Autodesk Inventor part; units mm, degrees
(part 2 of 3)
  spline S51 degree 3 poles (0.0984, 19.7366) (0.1649, 19.7419) (0.2979, 19.7525) (0.4939, 19.7932) (0.6876, 19.8429) (0.9422, 19.9224) (1.2539, 20.0412) (1.6171, 20.2089) (1.9698, 20.3977) (2.3118, 20.6053) (2.6441, 20.8281) (2.8566, 20.9892) (2.9629, 21.0697) knots 0 0 0 0 0.062465 0.124964 0.187468 0.249973 0.374966 0.499967 0.624972 0.749981 0.874991 1 1 1 1 construction
  arc A14 (2.9629, 21.0697) -> (2.8257, 22.375) centre (-14, 19.9467) ccw construction
  spline S52 degree 3 poles (2.8257, 22.375) (2.705, 22.4317) (2.4637, 22.545) (2.0923, 22.6939) (1.7146, 22.8258) (1.3304, 22.9372) (0.9402, 23.0257) (0.6106, 23.0771) (0.3451, 23.1019) (0.1453, 23.1102) (-0.055, 23.1093) (-0.1872, 23.092) (-0.2533, 23.0834) knots 0 0 0 0 0.125009 0.250019 0.375028 0.500033 0.625034 0.750027 0.812532 0.875036 0.937535 1 1 1 1 construction
  spline S53 degree 3 poles (-0.2533, 23.0834) (-0.3447, 23.0601) (-0.4818, 23.0252) (-0.668, 22.9946) (-0.8088, 22.9816) (-0.9502, 22.9756) (-1.0916, 22.9828) (-1.2322, 22.9989) (-1.3703, 23.0305) (-1.5044, 23.0763) (-1.6319, 23.1382) (-1.7501, 23.2166) (-1.8562, 23.3108) (-1.9467, 23.42) (-2.0197, 23.5419) (-2.07, 23.6744) (-2.1108, 23.8097) (-2.1574, 23.9432) (-2.1945, 24.08) (-2.2071, 24.2214) (-2.1981, 24.363) (-2.1676, 24.5016) (-2.118, 24.6344) (-2.0513, 24.7595) (-1.9698, 24.8754) (-1.8766, 24.9821) (-1.7723, 25.0778) (-1.6621, 25.1667) (-1.5442, 25.2449) (-1.4226, 25.3172) (-1.254, 25.4019) (-1.1226, 25.4542) (-1.035, 25.4891) knots 0 0 0 0 0.062498 0.093754 0.125008 0.156267 0.187517 0.21877 0.250029 0.281282 0.312529 0.343776 0.37503 0.406277 0.437515 0.468744 0.5 0.531256 0.562485 0.593723 0.62497 0.656224 0.687471 0.718718 0.749971 0.78123 0.812483 0.843733 0.874992 0.906246 0.937502 1 1 1 1 construction
  spline S54 degree 3 poles (-1.035, 25.4891) (-0.9764, 25.521) (-0.8593, 25.5847) (-0.6967, 25.7017) (-0.54, 25.8259) (-0.3398, 26.002) (-0.1033, 26.2373) (0.1603, 26.5383) (0.4057, 26.8542) (0.6337, 27.1829) (0.8467, 27.5217) (0.9753, 27.7552) (1.0396, 27.872) knots 0 0 0 0 0.062465 0.124964 0.187468 0.249973 0.374966 0.499967 0.624972 0.749981 0.874991 1 1 1 1 construction
  arc A15 (1.0396, 27.872) -> (0.3833, 29.0087) centre (-14, 19.9467) ccw construction
  spline S55 degree 3 poles (0.3833, 29.0087) (0.25, 29.0114) (-0.0165, 29.0168) (-0.4164, 29.0017) (-0.815, 28.9686) (-1.2114, 28.9141) (-1.6038, 28.8362) (-1.9258, 28.7491) (-2.1785, 28.6638) (-2.3644, 28.5901) (-2.5469, 28.5079) (-2.6607, 28.4383) (-2.7176, 28.4035) knots 0 0 0 0 0.125009 0.250019 0.375028 0.500033 0.625034 0.750027 0.812532 0.875036 0.937535 1 1 1 1 construction
  spline S56 degree 3 poles (-2.7176, 28.4035) (-2.7916, 28.3451) (-2.9027, 28.2574) (-3.0603, 28.1537) (-3.1837, 28.0846) (-3.3104, 28.0216) (-3.4424, 27.9706) (-3.5775, 27.9282) (-3.7165, 27.9008) (-3.8576, 27.8882) (-3.9993, 27.8929) (-4.1391, 27.9164) (-4.2744, 27.9593) (-4.4015, 28.0223) (-4.5177, 28.1039) (-4.6176, 28.2045) (-4.7099, 28.3115) (-4.8067, 28.4145) (-4.8963, 28.5244) (-4.9653, 28.6485) (-5.0147, 28.7815) (-5.0432, 28.9205) (-5.052, 29.062) (-5.0418, 29.2034) (-5.0145, 29.3424) (-4.9728, 29.4778) (-4.9164, 29.6077) (-4.852, 29.7336) (-4.7761, 29.8531) (-4.6944, 29.9686) (-4.5748, 30.1145) (-4.476, 30.2158) (-4.4102, 30.2833) knots 0 0 0 0 0.062498 0.093754 0.125008 0.156267 0.187517 0.21877 0.250029 0.281282 0.312529 0.343776 0.37503 0.406277 0.437515 0.468744 0.5 0.531256 0.562485 0.593723 0.62497 0.656224 0.687471 0.718718 0.749971 0.78123 0.812483 0.843733 0.874992 0.906246 0.937502 1 1 1 1 construction
  spline S57 degree 3 poles (-4.4102, 30.2833) (-4.3696, 30.3362) (-4.2885, 30.4421) (-4.1876, 30.6151) (-4.095, 30.7923) (-3.9837, 31.0346) (-3.8634, 31.3457) (-3.745, 31.7279) (-3.6493, 32.1164) (-3.5747, 32.5094) (-3.5179, 32.9054) (-3.4954, 33.1711) (-3.4842, 33.304) knots 0 0 0 0 0.062465 0.124964 0.187468 0.249973 0.374966 0.499967 0.624972 0.749981 0.874991 1 1 1 1 construction
  arc A16 (-3.4842, 33.304) -> (-4.546, 34.0754) centre (-14, 19.9467) ccw construction
  spline S58 degree 3 poles (-4.546, 34.0754) (-4.6689, 34.0237) (-4.9146, 33.9202) (-5.2737, 33.7438) (-5.6245, 33.5514) (-5.9644, 33.3404) (-6.2912, 33.1097) (-6.55, 32.8991) (-6.7461, 32.7184) (-6.8859, 32.5755) (-7.0193, 32.4261) (-7.0949, 32.3162) (-7.1327, 32.2613) knots 0 0 0 0 0.125009 0.250019 0.375028 0.500033 0.625034 0.750027 0.812532 0.875036 0.937535 1 1 1 1 construction
  spline S59 degree 3 poles (-7.1327, 32.2613) (-7.1766, 32.1779) (-7.2424, 32.0526) (-7.3442, 31.8938) (-7.4288, 31.7804) (-7.5189, 31.6713) (-7.6188, 31.5711) (-7.7249, 31.4773) (-7.8408, 31.3958) (-7.9646, 31.3269) (-8.0959, 31.2736) (-8.2332, 31.2381) (-8.3742, 31.2223) (-8.516, 31.2282) (-8.6553, 31.2555) (-8.7875, 31.3067) (-8.9154, 31.3669) (-9.0457, 31.4216) (-9.1722, 31.4856) (-9.2858, 31.5709) (-9.3849, 31.6723) (-9.4676, 31.7877) (-9.5331, 31.9134) (-9.5814, 32.0467) (-9.6129, 32.1848) (-9.6299, 32.3255) (-9.6312, 32.467) (-9.6236, 32.6084) (-9.6028, 32.7484) (-9.5752, 32.8871) (-9.5253, 33.069) (-9.4762, 33.2017) (-9.4436, 33.2902) knots 0 0 0 0 0.062498 0.093754 0.125008 0.156267 0.187517 0.21877 0.250029 0.281282 0.312529 0.343776 0.37503 0.406277 0.437515 0.468744 0.5 0.531256 0.562485 0.593723 0.62497 0.656224 0.687471 0.718718 0.749971 0.78123 0.812483 0.843733 0.874992 0.906246 0.937502 1 1 1 1 construction
  spline S60 degree 3 poles (-9.4436, 33.2902) (-9.428, 33.355) (-9.397, 33.4847) (-9.3752, 33.6838) (-9.3626, 33.8833) (-9.3595, 34.15) (-9.3762, 34.4832) (-9.4234, 34.8805) (-9.494, 35.2743) (-9.5857, 35.6636) (-9.695, 36.0485) (-9.7825, 36.3004) (-9.8262, 36.4263) knots 0 0 0 0 0.062465 0.124964 0.187468 0.249973 0.374966 0.499967 0.624972 0.749981 0.874991 1 1 1 1 construction
  arc A17 (-9.8262, 36.4263) -> (-11.11, 36.6992) centre (-14, 19.9467) ccw construction
  spline S61 degree 3 poles (-11.11, 36.6992) (-11.2012, 36.602) (-11.3836, 36.4075) (-11.64, 36.1003) (-11.8821, 35.7819) (-12.1068, 35.4508) (-12.3116, 35.1071) (-12.4623, 34.8095) (-12.5679, 34.5647) (-12.6376, 34.3772) (-12.6986, 34.1865) (-12.723, 34.0554) (-12.7352, 33.9898) knots 0 0 0 0 0.125009 0.250019 0.375028 0.500033 0.625034 0.750027 0.812532 0.875036 0.937535 1 1 1 1 construction
  spline S62 degree 3 poles (-12.7352, 33.9898) (-12.7413, 33.8958) (-12.7505, 33.7546) (-12.7789, 33.5681) (-12.8101, 33.4301) (-12.8481, 33.2938) (-12.8986, 33.1615) (-12.9574, 33.0328) (-13.0301, 32.9112) (-13.1151, 32.7978) (-13.2134, 32.6957) (-13.3244, 32.6075) (-13.4468, 32.5357) (-13.5787, 32.4834) (-13.7171, 32.4516) (-13.8587, 32.4447) (-14, 32.4477) (-14.1413, 32.4447) (-14.2829, 32.4516) (-14.4213, 32.4834) (-14.5532, 32.5357) (-14.6756, 32.6075) (-14.7866, 32.6957) (-14.8849, 32.7978) (-14.9699, 32.9112) (-15.0426, 33.0328) (-15.1014, 33.1615) (-15.1519, 33.2938) (-15.1899, 33.4301) (-15.2211, 33.5681) (-15.2495, 33.7546) (-15.2587, 33.8958) (-15.2648, 33.9898) knots 0 0 0 0 0.062498 0.093754 0.125008 0.156267 0.187517 0.21877 0.250029 0.281282 0.312529 0.343776 0.37503 0.406277 0.437515 0.468744 0.5 0.531256 0.562485 0.593723 0.62497 0.656224 0.687471 0.718718 0.749971 0.78123 0.812483 0.843733 0.874992 0.906246 0.937502 1 1 1 1 construction
  spline S63 degree 3 poles (-15.2648, 33.9898) (-15.277, 34.0554) (-15.3014, 34.1865) (-15.3624, 34.3772) (-15.4321, 34.5647) (-15.5377, 34.8095) (-15.6884, 35.1071) (-15.8932, 35.4508) (-16.1179, 35.7819) (-16.36, 36.1003) (-16.6164, 36.4075) (-16.7988, 36.602) (-16.89, 36.6992) knots 0 0 0 0 0.062465 0.124964 0.187468 0.249973 0.374966 0.499967 0.624972 0.749981 0.874991 1 1 1 1 construction
  arc A18 (-16.89, 36.6992) -> (-18.1738, 36.4263) centre (-14, 19.9467) ccw construction
  circle A19 centre (-14, 19.9467) radius 1.1 construction
  spline S64 degree 3 poles (-41.4547, 4.7129) (-41.4384, 4.8452) (-41.4058, 5.1098) (-41.3799, 5.5091) (-41.3721, 5.9091) (-41.3859, 6.3089) (-41.4232, 6.7073) (-41.477, 7.0365) (-41.5361, 7.2965) (-41.5904, 7.489) (-41.6536, 7.679) (-41.7112, 7.7993) (-41.74, 7.8594) knots 0 0 0 0 0.125009 0.250019 0.375028 0.500033 0.625034 0.750027 0.812532 0.875036 0.937535 1 1 1 1 construction
  spline S65 degree 3 poles (-41.74, 7.8594) (-41.7905, 7.939) (-41.8663, 8.0584) (-41.9534, 8.2258) (-42.0096, 8.3556) (-42.0593, 8.4881) (-42.0965, 8.6247) (-42.125, 8.7634) (-42.1379, 8.9044) (-42.1361, 9.0461) (-42.117, 9.1866) (-42.0793, 9.3233) (-42.0228, 9.4534) (-41.9472, 9.5734) (-41.8541, 9.6807) (-41.7438, 9.7698) (-41.6279, 9.8507) (-41.5156, 9.9365) (-41.3972, 10.0144) (-41.2666, 10.0704) (-41.1293, 10.1059) (-40.9881, 10.1201) (-40.8464, 10.1143) (-40.7068, 10.0898) (-40.5713, 10.0484) (-40.4409, 9.9931) (-40.3175, 9.9238) (-40.1987, 9.8467) (-40.0876, 9.759) (-39.9811, 9.666) (-39.8482, 9.5321) (-39.7575, 9.4235) (-39.6971, 9.3511) knots 0 0 0 0 0.062498 0.093754 0.125008 0.156267 0.187517 0.21877 0.250029 0.281282 0.312529 0.343776 0.37503 0.406277 0.437515 0.468744 0.5 0.531256 0.562485 0.593723 0.62497 0.656224 0.687471 0.718718 0.749971 0.78123 0.812483 0.843733 0.874992 0.906246 0.937502 1 1 1 1 construction
  spline S66 degree 3 poles (-39.6971, 9.3511) (-39.6486, 9.3054) (-39.5515, 9.2139) (-39.3897, 9.0958) (-39.223, 8.9856) (-38.9932, 8.8501) (-38.6961, 8.6987) (-38.328, 8.5418) (-37.9513, 8.4069) (-37.568, 8.2926) (-37.1798, 8.1957) (-36.9178, 8.1462) (-36.7868, 8.1214) knots 0 0 0 0 0.062465 0.124964 0.187468 0.249973 0.374966 0.499967 0.624972 0.749981 0.874991 1 1 1 1 construction
  arc A20 (-36.7868, 8.1214) -> (-35.9109, 9.0989) centre (-49, 19.9467) ccw construction
  spline S67 degree 3 poles (-35.9109, 9.0989) (-35.9498, 9.2264) (-36.0277, 9.4814) (-36.1664, 9.8567) (-36.322, 10.2252) (-36.4972, 10.5849) (-36.6933, 10.9336) (-36.8763, 11.2125) (-37.0361, 11.426) (-37.1639, 11.5798) (-37.299, 11.7277) (-37.4005, 11.8141) (-37.4513, 11.8573) knots 0 0 0 0 0.125009 0.250019 0.375028 0.500033 0.625034 0.750027 0.812532 0.875036 0.937535 1 1 1 1 construction
  spline S68 degree 3 poles (-37.4513, 11.8573) (-37.5298, 11.9095) (-37.6477, 11.9877) (-37.7953, 12.1053) (-37.8994, 12.201) (-37.9987, 12.3018) (-38.0883, 12.4114) (-38.1707, 12.5265) (-38.2399, 12.6501) (-38.2959, 12.7803) (-38.3355, 12.9164) (-38.3567, 13.0566) (-38.358, 13.1985) (-38.3377, 13.3389) (-38.2963, 13.4748) (-38.2319, 13.601) (-38.1589, 13.7221) (-38.0912, 13.8461) (-38.0146, 13.9654) (-37.9182, 14.0697) (-37.8071, 14.158) (-37.6839, 14.2284) (-37.5522, 14.2807) (-37.4146, 14.3151) (-37.274, 14.3324) (-37.1324, 14.3349) (-36.9914, 14.3218) (-36.8516, 14.2997) (-36.7145, 14.2648) (-36.5793, 14.2231) (-36.4034, 14.1549) (-36.2764, 14.0925) (-36.1918, 14.051) knots 0 0 0 0 0.062498 0.093754 0.125008 0.156267 0.187517 0.21877 0.250029 0.281282 0.312529 0.343776 0.37503 0.406277 0.437515 0.468744 0.5 0.531256 0.562485 0.593723 0.62497 0.656224 0.687471 0.718718 0.749971 0.78123 0.812483 0.843733 0.874992 0.906246 0.937502 1 1 1 1 construction
  spline S69 degree 3 poles (-36.1918, 14.051) (-36.1288, 14.0289) (-36.003, 13.9848) (-35.8072, 13.9428) (-35.61, 13.9099) (-35.345, 13.8796) (-35.0119, 13.8621) (-34.6118, 13.8685) (-34.2129, 13.8985) (-33.8162, 13.95) (-33.4221, 14.0193) (-33.1626, 14.0806) (-33.0329, 14.1113) knots 0 0 0 0 0.062465 0.124964 0.187468 0.249973 0.374966 0.499967 0.624972 0.749981 0.874991 1 1 1 1 construction
  arc A21 (-33.0329, 14.1113) -> (-32.6303, 15.3605) centre (-49, 19.9467) ccw construction
  spline S70 degree 3 poles (-32.6303, 15.3605) (-32.7177, 15.4612) (-32.8926, 15.6625) (-33.172, 15.9489) (-33.464, 16.2223) (-33.7703, 16.4796) (-34.0914, 16.7184) (-34.372, 16.8987) (-34.6048, 17.0288) (-34.7841, 17.1173) (-34.9676, 17.1975) (-35.0955, 17.2352) (-35.1595, 17.254) knots 0 0 0 0 0.125009 0.250019 0.375028 0.500033 0.625034 0.750027 0.812532 0.875036 0.937535 1 1 1 1 construction
  spline S71 degree 3 poles (-35.1595, 17.254) (-35.2525, 17.2697) (-35.3919, 17.2932) (-35.5746, 17.3405) (-35.7087, 17.3857) (-35.8404, 17.4374) (-35.9668, 17.5011) (-36.0889, 17.5727) (-36.2024, 17.6575) (-36.3065, 17.7536) (-36.398, 17.8619) (-36.4744, 17.9813) (-36.5333, 18.1104) (-36.5719, 18.2469) (-36.5893, 18.3879) (-36.5818, 18.5294) (-36.5644, 18.6697) (-36.553, 18.8105) (-36.5316, 18.9507) (-36.4858, 19.0851) (-36.4203, 19.211) (-36.3364, 19.3254) (-36.2373, 19.4268) (-36.1257, 19.5142) (-36.0043, 19.5872) (-35.8759, 19.6471) (-35.7418, 19.6924) (-35.6051, 19.7291) (-35.4656, 19.753) (-35.3251, 19.7699) (-35.1367, 19.7791) (-34.9953, 19.7738) (-34.9011, 19.7703) knots 0 0 0 0 0.062498 0.093754 0.125008 0.156267 0.187517 0.21877 0.250029 0.281282 0.312529 0.343776 0.37503 0.406277 0.437515 0.468744 0.5 0.531256 0.562485 0.593723 0.62497 0.656224 0.687471 0.718718 0.749971 0.78123 0.812483 0.843733 0.874992 0.906246 0.937502 1 1 1 1 construction
  spline S72 degree 3 poles (-34.9011, 19.7703) (-34.8347, 19.7757) (-34.7017, 19.7866) (-34.5057, 19.8279) (-34.3122, 19.878) (-34.0578, 19.9581) (-33.7464, 20.0776) (-33.3836, 20.2462) (-33.0313, 20.4359) (-32.6898, 20.6442) (-32.358, 20.8679) (-32.1459, 21.0294) (-32.0399, 21.1102) knots 0 0 0 0 0.062465 0.124964 0.187468 0.249973 0.374966 0.499967 0.624972 0.749981 0.874991 1 1 1 1 construction
  arc A22 (-32.0399, 21.1102) -> (-32.1802, 22.4152) centre (-49, 19.9467) ccw construction
  spline S73 degree 3 poles (-32.1802, 22.4152) (-32.301, 22.4716) (-32.5426, 22.5844) (-32.9143, 22.7323) (-33.2923, 22.8633) (-33.6768, 22.9738) (-34.0672, 23.0614) (-34.3969, 23.112) (-34.6625, 23.1362) (-34.8623, 23.144) (-35.0626, 23.1426) (-35.1948, 23.125) (-35.2609, 23.1162) knots 0 0 0 0 0.125009 0.250019 0.375028 0.500033 0.625034 0.750027 0.812532 0.875036 0.937535 1 1 1 1 construction
  spline S74 degree 3 poles (-35.2609, 23.1162) (-35.3522, 23.0927) (-35.4892, 23.0575) (-35.6753, 23.0265) (-35.8161, 23.0131) (-35.9575, 23.0068) (-36.0989, 23.0136) (-36.2395, 23.0294) (-36.3777, 23.0606) (-36.5119, 23.1062) (-36.6395, 23.1678) (-36.7579, 23.2458) (-36.8643, 23.3398) (-36.955, 23.4488) (-37.0283, 23.5705) (-37.079, 23.7029) (-37.1201, 23.8381) (-37.167, 23.9714) (-37.2044, 24.1082) (-37.2173, 24.2496) (-37.2087, 24.3912) (-37.1785, 24.5299) (-37.1293, 24.6628) (-37.0628, 24.788) (-36.9816, 24.9041) (-36.8886, 25.0111) (-36.7846, 25.107) (-36.6746, 25.1961) (-36.5569, 25.2747) (-36.4355, 25.3473) (-36.2671, 25.4323) (-36.1358, 25.485) (-36.0483, 25.5201) knots 0 0 0 0 0.062498 0.093754 0.125008 0.156267 0.187517 0.21877 0.250029 0.281282 0.312529 0.343776 0.37503 0.406277 0.437515 0.468744 0.5 0.531256 0.562485 0.593723 0.62497 0.656224 0.687471 0.718718 0.749971 0.78123 0.812483 0.843733 0.874992 0.906246 0.937502 1 1 1 1 construction
  spline S75 degree 3 poles (-36.0483, 25.5201) (-35.9898, 25.5521) (-35.8728, 25.6161) (-35.7105, 25.7335) (-35.5541, 25.858) (-35.3543, 26.0346) (-35.1184, 26.2705) (-34.8555, 26.5721) (-34.6108, 26.8886) (-34.3836, 27.2179) (-34.1715, 27.5571) (-34.0434, 27.791) (-33.9794, 27.9079) knots 0 0 0 0 0.062465 0.124964 0.187468 0.249973 0.374966 0.499967 0.624972 0.749981 0.874991 1 1 1 1 construction
  arc A23 (-33.9794, 27.9079) -> (-34.6384, 29.043) centre (-49, 19.9467) ccw construction
  spline S76 degree 3 poles (-34.6384, 29.043) (-34.7717, 29.0454) (-35.0383, 29.0501) (-35.438, 29.0341) (-35.8366, 29.0001) (-36.2328, 28.9446) (-36.6251, 28.8658) (-36.9469, 28.7779) (-37.1993, 28.692) (-37.385, 28.6179) (-37.5674, 28.5352) (-37.681, 28.4653) (-37.7378, 28.4304) knots 0 0 0 0 0.125009 0.250019 0.375028 0.500033 0.625034 0.750027 0.812532 0.875036 0.937535 1 1 1 1 construction
  spline S77 degree 3 poles (-37.7378, 28.4304) (-37.8117, 28.3718) (-37.9225, 28.2839) (-38.0799, 28.1798) (-38.2032, 28.1104) (-38.3297, 28.0471) (-38.4616, 27.9958) (-38.5966, 27.953) (-38.7355, 27.9254) (-38.8766, 27.9124) (-39.0183, 27.9168) (-39.1582, 27.9399) (-39.2935, 27.9825) (-39.4208, 28.0452) (-39.5372, 28.1265) (-39.6374, 28.2268) (-39.73, 28.3337) (-39.827, 28.4364) (-39.9168, 28.5461) (-39.9861, 28.67) (-40.0358, 28.8029) (-40.0647, 28.9418) (-40.0738, 29.0833) (-40.064, 29.2248) (-40.037, 29.3638) (-39.9956, 29.4993) (-39.9396, 29.6293) (-39.8754, 29.7555) (-39.7998, 29.8751) (-39.7184, 29.9908) (-39.5991, 30.137) (-39.5006, 30.2385) (-39.4349, 30.3062) knots 0 0 0 0 0.062498 0.093754 0.125008 0.156267 0.187517 0.21877 0.250029 0.281282 0.312529 0.343776 0.37503 0.406277 0.437515 0.468744 0.5 0.531256 0.562485 0.593723 0.62497 0.656224 0.687471 0.718718 0.749971 0.78123 0.812483 0.843733 0.874992 0.906246 0.937502 1 1 1 1 construction
  spline S78 degree 3 poles (-39.4349, 30.3062) (-39.3945, 30.3592) (-39.3136, 30.4653) (-39.2132, 30.6385) (-39.1209, 30.8159) (-39.0102, 31.0585) (-38.8907, 31.3699) (-38.7731, 31.7524) (-38.6784, 32.1411) (-38.6048, 32.5343) (-38.5489, 32.9305) (-38.5271, 33.1962) (-38.5161, 33.3291) knots 0 0 0 0 0.062465 0.124964 0.187468 0.249973 0.374966 0.499967 0.624972 0.749981 0.874991 1 1 1 1 construction
  arc A24 (-38.5161, 33.3291) -> (-39.5798, 34.098) centre (-49, 19.9467) ccw construction
  spline S79 degree 3 poles (-39.5798, 34.098) (-39.7025, 34.046) (-39.948, 33.9419) (-40.3067, 33.7646) (-40.657, 33.5714) (-40.9964, 33.3595) (-41.3227, 33.128) (-41.5809, 32.9169) (-41.7766, 32.7357) (-41.9161, 32.5925) (-42.0491, 32.4427) (-42.1245, 32.3327) (-42.1621, 32.2777) knots 0 0 0 0 0.125009 0.250019 0.375028 0.500033 0.625034 0.750027 0.812532 0.875036 0.937535 1 1 1 1 construction
  spline S80 degree 3 poles (-42.1621, 32.2777) (-42.2058, 32.1941) (-42.2713, 32.0687) (-42.3727, 31.9096) (-42.4571, 31.7961) (-42.547, 31.6868) (-42.6466, 31.5863) (-42.7525, 31.4923) (-42.8682, 31.4105) (-42.9918, 31.3413) (-43.123, 31.2876) (-43.2602, 31.2519) (-43.4012, 31.2357) (-43.5429, 31.2412) (-43.6824, 31.2682) (-43.8147, 31.3191) (-43.9427, 31.379) (-44.0731, 31.4334) (-44.1998, 31.4971) (-44.3135, 31.5821) (-44.413, 31.6833) (-44.4959, 31.7985) (-44.5617, 31.9241) (-44.6103, 32.0572) (-44.6422, 32.1953) (-44.6595, 32.3359) (-44.6612, 32.4774) (-44.6538, 32.6188) (-44.6334, 32.7588) (-44.6061, 32.8976) (-44.5566, 33.0797) (-44.5079, 33.2125) (-44.4754, 33.301) knots 0 0 0 0 0.062498 0.093754 0.125008 0.156267 0.187517 0.21877 0.250029 0.281282 0.312529 0.343776 0.37503 0.406277 0.437515 0.468744 0.5 0.531256 0.562485 0.593723 0.62497 0.656224 0.687471 0.718718 0.749971 0.78123 0.812483 0.843733 0.874992 0.906246 0.937502 1 1 1 1 construction
  spline S81 degree 3 poles (-44.4754, 33.301) (-44.4601, 33.3659) (-44.4294, 33.4957) (-44.408, 33.6948) (-44.3959, 33.8944) (-44.3935, 34.1611) (-44.4109, 34.4942) (-44.4591, 34.8913) (-44.5306, 35.285) (-44.6233, 35.6741) (-44.7334, 36.0588) (-44.8216, 36.3104) (-44.8656, 36.4363) knots 0 0 0 0 0.062465 0.124964 0.187468 0.249973 0.374966 0.499967 0.624972 0.749981 0.874991 1 1 1 1 construction
  arc A25 (-44.8656, 36.4363) -> (-46.1501, 36.7061) centre (-49, 19.9467) ccw construction
  spline S82 degree 3 poles (-46.1501, 36.7061) (-46.241, 36.6086) (-46.423, 36.4137) (-46.6786, 36.1059) (-46.92, 35.7869) (-47.1438, 35.4553) (-47.3478, 35.1111) (-47.4978, 34.8132) (-47.6028, 34.568) (-47.6721, 34.3805) (-47.7326, 34.1896) (-47.7567, 34.0584) (-47.7688, 33.9928) knots 0 0 0 0 0.125009 0.250019 0.375028 0.500033 0.625034 0.750027 0.812532 0.875036 0.937535 1 1 1 1 construction
  spline S83 degree 3 poles (-47.7688, 33.9928) (-47.7747, 33.8987) (-47.7835, 33.7575) (-47.8115, 33.5709) (-47.8423, 33.4329) (-47.88, 33.2965) (-47.9301, 33.1641) (-47.9886, 33.0352) (-48.0611, 32.9134) (-48.1458, 32.7999) (-48.2439, 32.6975) (-48.3547, 32.6091) (-48.4769, 32.537) (-48.6086, 32.4844) (-48.747, 32.4523) (-48.8886, 32.445) (-49.0299, 32.4476) (-49.1712, 32.4443) (-49.3128, 32.4509) (-49.4513, 32.4823) (-49.5833, 32.5343) (-49.7058, 32.6058) (-49.8171, 32.6938) (-49.9156, 32.7957) (-50.0009, 32.9088) (-50.0739, 33.0302) (-50.133, 33.1589) (-50.1838, 33.291) (-50.2221, 33.4272) (-50.2536, 33.5651) (-50.2825, 33.7516) (-50.292, 33.8927) (-50.2983, 33.9868) knots 0 0 0 0 0.062498 0.093754 0.125008 0.156267 0.187517 0.21877 0.250029 0.281282 0.312529 0.343776 0.37503 0.406277 0.437515 0.468744 0.5 0.531256 0.562485 0.593723 0.62497 0.656224 0.687471 0.718718 0.749971 0.78123 0.812483 0.843733 0.874992 0.906246 0.937502 1 1 1 1 construction
  spline S84 degree 3 poles (-50.2983, 33.9868) (-50.3107, 34.0523) (-50.3354, 34.1834) (-50.3969, 34.3739) (-50.467, 34.5612) (-50.5732, 34.8058) (-50.7246, 35.103) (-50.9302, 35.4463) (-51.1557, 35.7768) (-51.3986, 36.0946) (-51.6557, 36.4012) (-51.8385, 36.5952) (-51.93, 36.6923) knots 0 0 0 0 0.062465 0.124964 0.187468 0.249973 0.374966 0.499967 0.624972 0.749981 0.874991 1 1 1 1 construction
  arc A26 (-51.93, 36.6923) -> (-53.2131, 36.4163) centre (-49, 19.9467) ccw construction
  spline S85 degree 3 poles (-53.2131, 36.4163) (-53.2566, 36.2903) (-53.3435, 36.0382) (-53.4518, 35.653) (-53.5426, 35.2635) (-53.6122, 34.8695) (-53.6586, 34.4721) (-53.6744, 34.1389) (-53.6707, 33.8722) (-53.6576, 33.6727) (-53.6353, 33.4737) (-53.604, 33.3441) (-53.5883, 33.2793) knots 0 0 0 0 0.125009 0.250019 0.375028 0.500033 0.625034 0.750027 0.812532 0.875036 0.937535 1 1 1 1 construction
  spline S86 degree 3 poles (-53.5883, 33.2793) (-53.5554, 33.1909) (-53.5061, 33.0583) (-53.4557, 32.8765) (-53.4278, 32.7378) (-53.4067, 32.5979) (-53.3987, 32.4566) (-53.3997, 32.315) (-53.4163, 32.1743) (-53.4475, 32.0361) (-53.4955, 31.9027) (-53.5607, 31.7768) (-53.6431, 31.6613) (-53.742, 31.5596) (-53.8554, 31.474) (-53.9817, 31.4098) (-54.1119, 31.3547) (-54.2396, 31.2942) (-54.3717, 31.2427) (-54.511, 31.215) (-54.6527, 31.2089) (-54.7937, 31.2243) (-54.9311, 31.2594) (-55.0626, 31.3124) (-55.1865, 31.3811) (-55.3026, 31.4623) (-55.4089, 31.5558) (-55.5091, 31.6558) (-55.5995, 31.7647) (-55.6843, 31.8778) (-55.7865, 32.0365) (-55.8526, 32.1615) (-55.8967, 32.2449) knots 0 0 0 0 0.062498 0.093754 0.125008 0.156267 0.187517 0.21877 0.250029 0.281282 0.312529 0.343776 0.37503 0.406277 0.437515 0.468744 0.5 0.531256 0.562485 0.593723 0.62497 0.656224 0.687471 0.718718 0.749971 0.78123 0.812483 0.843733 0.874992 0.906246 0.937502 1 1 1 1 construction
  spline S87 degree 3 poles (-55.8967, 32.2449) (-55.9346, 32.2997) (-56.0105, 32.4094) (-56.1442, 32.5585) (-56.2844, 32.701) (-56.481, 32.8813) (-56.7402, 33.0912) (-57.0676, 33.3212) (-57.408, 33.5314) (-57.7592, 33.7229) (-58.1187, 33.8985) (-58.3647, 34.0014) (-58.4877, 34.0528) knots 0 0 0 0 0.062465 0.124964 0.187468 0.249973 0.374966 0.499967 0.624972 0.749981 0.874991 1 1 1 1 construction
  arc A27 (-58.4877, 34.0528) -> (-59.5477, 33.2788) centre (-49, 19.9467) ccw construction
  spline S88 degree 3 poles (-59.5477, 33.2788) (-59.5361, 33.146) (-59.513, 32.8804) (-59.4553, 32.4845) (-59.3798, 32.0916) (-59.2831, 31.7034) (-59.1638, 31.3215) (-59.0428, 31.0107) (-58.9309, 30.7686) (-58.8378, 30.5916) (-58.7365, 30.4189) (-58.6551, 30.3132) (-58.6145, 30.2604) knots 0 0 0 0 0.125009 0.250019 0.375028 0.500033 0.625034 0.750027 0.812532 0.875036 0.937535 1 1 1 1 construction
  spline S89 degree 3 poles (-58.6145, 30.2604) (-58.5485, 30.193) (-58.4495, 30.092) (-58.3295, 29.9463) (-58.2476, 29.831) (-58.1714, 29.7118) (-58.1066, 29.5859) (-58.0499, 29.4562) (-58.0079, 29.3209) (-57.9803, 29.182) (-57.9698, 29.0406) (-57.9782, 28.899) (-58.0064, 28.76) (-58.0554, 28.6269) (-58.1242, 28.5026) (-58.2135, 28.3925) (-58.31, 28.2893) (-58.4021, 28.182) (-58.5018, 28.0812) (-58.6178, 27.9993) (-58.7447, 27.936) (-58.8799, 27.8928) (-59.0197, 27.869) (-59.1613, 27.8639) (-59.3025, 27.8762) (-59.4416, 27.9032) (-59.5767, 27.9454) (-59.7088, 27.996) (-59.8357, 28.0587) (-59.9593, 28.1276) (-60.1172, 28.2309) (-60.2284, 28.3183) (-60.3026, 28.3765) knots 0 0 0 0 0.062498 0.093754 0.125008 0.156267 0.187517 0.21877 0.250029 0.281282 0.312529 0.343776 0.37503 0.406277 0.437515 0.468744 0.5 0.531256 0.562485 0.593723 0.62497 0.656224 0.687471 0.718718 0.749971 0.78123 0.812483 0.843733 0.874992 0.906246 0.937502 1 1 1 1 construction
  spline S90 degree 3 poles (-60.3026, 28.3765) (-60.3595, 28.4112) (-60.4735, 28.4805) (-60.6563, 28.5623) (-60.8423, 28.6355) (-61.0952, 28.7203) (-61.4174, 28.8066) (-61.81, 28.8835) (-62.2065, 28.9371) (-62.6052, 28.9692) (-63.0051, 28.9833) (-63.2717, 28.9773) (-63.4049, 28.9743) knots 0 0 0 0 0.062465 0.124964 0.187468 0.249973 0.374966 0.499967 0.624972 0.749981 0.874991 1 1 1 1 construction
  arc A28 (-63.4049, 28.9743) -> (-64.0585, 27.8361) centre (-49, 19.9467) ccw construction
  spline S91 degree 3 poles (-64.0585, 27.8361) (-63.9939, 27.7194) (-63.8647, 27.4862) (-63.6509, 27.148) (-63.4222, 26.8198) (-63.176, 26.5044) (-62.9117, 26.2041) (-62.6747, 25.9694) (-62.474, 25.7937) (-62.317, 25.6699) (-62.1542, 25.5533) (-62.0369, 25.4898) (-61.9782, 25.4581) knots 0 0 0 0 0.125009 0.250019 0.375028 0.500033 0.625034 0.750027 0.812532 0.875036 0.937535 1 1 1 1 construction
  spline S92 degree 3 poles (-61.9782, 25.4581) (-61.8905, 25.4234) (-61.759, 25.3714) (-61.5902, 25.2872) (-61.4684, 25.2152) (-61.3503, 25.1372) (-61.2399, 25.0486) (-61.1354, 24.9531) (-61.042, 24.8466) (-60.9602, 24.7309) (-60.8931, 24.606) (-60.8432, 24.4733) (-60.8125, 24.3348) (-60.8031, 24.1932) (-60.8154, 24.0517) (-60.8521, 23.9148) (-60.8984, 23.7813) (-60.9388, 23.6459) (-60.9889, 23.5133) (-61.0616, 23.3912) (-61.1518, 23.2818) (-61.2577, 23.1873) (-61.3757, 23.1087) (-61.5031, 23.0465) (-61.637, 23.0003) (-61.7751, 22.9684) (-61.9157, 22.9519) (-62.057, 22.9444) (-62.1984, 22.9501) (-62.3393, 22.9627) (-62.5255, 22.9929) (-62.6627, 23.0275) (-62.7541, 23.0505) knots 0 0 0 0 0.062498 0.093754 0.125008 0.156267 0.187517 0.21877 0.250029 0.281282 0.312529 0.343776 0.37503 0.406277 0.437515 0.468744 0.5 0.531256 0.562485 0.593723 0.62497 0.656224 0.687471 0.718718 0.749971 0.78123 0.812483 0.843733 0.874992 0.906246 0.937502 1 1 1 1 construction
  spline S93 degree 3 poles (-62.7541, 23.0505) (-62.8203, 23.059) (-62.9525, 23.076) (-63.1528, 23.0764) (-63.3526, 23.0676) (-63.618, 23.0422) (-63.9475, 22.99) (-64.3375, 22.9005) (-64.7215, 22.7883) (-65.0988, 22.6554) (-65.4698, 22.5057) (-65.7109, 22.3918) (-65.8314, 22.3348) knots 0 0 0 0 0.062465 0.124964 0.187468 0.249973 0.374966 0.499967 0.624972 0.749981 0.874991 1 1 1 1 construction
  arc A29 (-65.8314, 22.3348) -> (-65.9655, 21.0292) centre (-49, 19.9467) ccw construction
  spline S94 degree 3 poles (-65.9655, 21.0292) (-65.8591, 20.9489) (-65.6462, 20.7883) (-65.3133, 20.5663) (-64.9709, 20.3596) (-64.6177, 20.1716) (-64.254, 20.0047) (-63.9421, 19.8867) (-63.6873, 19.8078) (-63.4935, 19.7586) (-63.2973, 19.7183) (-63.1644, 19.708) (-63.0979, 19.7029) knots 0 0 0 0 0.125009 0.250019 0.375028 0.500033 0.625034 0.750027 0.812532 0.875036 0.937535 1 1 1 1 construction
  spline S95 degree 3 poles (-63.0979, 19.7029) (-63.0037, 19.7069) (-62.8624, 19.7129) (-62.6739, 19.7046) (-62.5333, 19.6883) (-62.3937, 19.6651) (-62.2569, 19.6291) (-62.1226, 19.5844) (-61.9939, 19.5251) (-61.8721, 19.4527) (-61.7601, 19.3658) (-61.6605, 19.2649) (-61.576, 19.1509) (-61.5099, 19.0254) (-61.4635, 18.8911) (-61.4415, 18.7511) (-61.4294, 18.6103) (-61.4113, 18.4701) (-61.4031, 18.3286) (-61.4198, 18.1875) (-61.4577, 18.0508) (-61.516, 17.9215) (-61.5919, 17.8017) (-61.6829, 17.693) (-61.7865, 17.5964) (-61.8996, 17.5111) (-62.0214, 17.4388) (-62.1475, 17.3745) (-62.2789, 17.3222) (-62.4128, 17.2764) (-62.5952, 17.2282) (-62.7346, 17.204) (-62.8275, 17.1879) knots 0 0 0 0 0.062498 0.093754 0.125008 0.156267 0.187517 0.21877 0.250029 0.281282 0.312529 0.343776 0.37503 0.406277 0.437515 0.468744 0.5 0.531256 0.562485 0.593723 0.62497 0.656224 0.687471 0.718718 0.749971 0.78123 0.812483 0.843733 0.874992 0.906246 0.937502 1 1 1 1 construction
  spline S96 degree 3 poles (-62.8275, 17.1879) (-62.8913, 17.1687) (-63.0191, 17.1304) (-63.2022, 17.0494) (-63.3811, 16.9601) (-63.6133, 16.8289) (-63.893, 16.6472) (-64.2129, 16.4069) (-64.5181, 16.1481) (-64.8087, 15.8733) (-65.0868, 15.5856) (-65.2607, 15.3834) (-65.3476, 15.2824) knots 0 0 0 0 0.062465 0.124964 0.187468 0.249973 0.374966 0.499967 0.624972 0.749981 0.874991 1 1 1 1 construction
  arc A30 (-65.3476, 15.2824) -> (-64.939, 14.0351) centre (-49, 19.9467) ccw construction
  spline S97 degree 3 poles (-64.939, 14.0351) (-64.8091, 14.005) (-64.5494, 13.9449) (-64.155, 13.8775) (-63.7581, 13.8279) (-63.3589, 13.7998) (-62.9589, 13.7953) (-62.6259, 13.8144) (-62.361, 13.846) (-62.164, 13.8798) (-61.9684, 13.9228) (-61.8427, 13.9675) (-61.7799, 13.9899) knots 0 0 0 0 0.125009 0.250019 0.375028 0.500033 0.625034 0.750027 0.812532 0.875036 0.937535 1 1 1 1 construction
  spline S98 degree 3 poles (-61.7799, 13.9899) (-61.6955, 14.0318) (-61.5688, 14.0947) (-61.3932, 14.1638) (-61.2582, 14.2061) (-61.1213, 14.2417) (-60.9816, 14.2645) (-60.8407, 14.2783) (-60.699, 14.2764) (-60.5583, 14.2598) (-60.4206, 14.2261) (-60.2886, 14.1743) (-60.1651, 14.1045) (-60.0536, 14.0168) (-59.9567, 13.913) (-59.8796, 13.794) (-59.8112, 13.6703) (-59.7377, 13.5496) (-59.6726, 13.4237) (-59.6306, 13.288) (-59.6096, 13.1477) (-59.6102, 13.0058) (-59.6308, 12.8655) (-59.6698, 12.7292) (-59.7251, 12.5988) (-59.7937, 12.4749) (-59.8756, 12.3594) (-59.9646, 12.2493) (-60.0634, 12.148) (-60.1671, 12.0518) (-60.3142, 11.9336) (-60.4316, 11.8548) (-60.5099, 11.8023) knots 0 0 0 0 0.062498 0.093754 0.125008 0.156267 0.187517 0.21877 0.250029 0.281282 0.312529 0.343776 0.37503 0.406277 0.437515 0.468744 0.5 0.531256 0.562485 0.593723 0.62497 0.656224 0.687471 0.718718 0.749971 0.78123 0.812483 0.843733 0.874992 0.906246 0.937502 1 1 1 1 construction
  spline S99 degree 3 poles (-60.5099, 11.8023) (-60.5605, 11.7588) (-60.6616, 11.6718) (-60.7959, 11.5233) (-60.923, 11.369) (-61.0818, 11.1547) (-61.2635, 10.8749) (-61.4579, 10.5252) (-61.6314, 10.1647) (-61.7852, 9.7954) (-61.9222, 9.4195) (-61.9988, 9.1641) (-62.0371, 9.0364) knots 0 0 0 0 0.062465 0.124964 0.187468 0.249973 0.374966 0.499967 0.624972 0.749981 0.874991 1 1 1 1 construction
  arc A31 (-62.0371, 9.0364) -> (-61.1566, 8.0632) centre (-49, 19.9467) ccw construction
  spline S100 degree 3 poles (-61.1566, 8.0632) (-61.0257, 8.0886) (-60.7639, 8.1393) (-60.3762, 8.2381) (-59.9934, 8.3543) (-59.6174, 8.491) (-59.2501, 8.6496) (-58.9536, 8.8024) (-58.7245, 8.939) (-58.5583, 9.05) (-58.3971, 9.1689) (-58.3005, 9.2608) (-58.2522, 9.3068) knots 0 0 0 0 0.125009 0.250019 0.375028 0.500033 0.625034 0.750027 0.812532 0.875036 0.937535 1 1 1 1 construction
  spline S101 degree 3 poles (-58.2522, 9.3068) (-58.1921, 9.3795) (-58.102, 9.4885) (-57.9697, 9.623) (-57.8636, 9.7166) (-57.7529, 9.8048) (-57.6346, 9.8824) (-57.5115, 9.9523) (-57.3813, 10.0082) (-57.246, 10.0503) (-57.1065, 10.0755) (-56.9648, 10.0819) (-56.8236, 10.0684) (-56.6861, 10.0335) (-56.5553, 9.9781) (-56.4365, 9.9009) (-56.3237, 9.8156) (-56.2074, 9.7353) (-56.0968, 9.6467) (-56.0032, 9.5399) (-55.927, 9.4202) (-55.8698, 9.2903) (-55.8316, 9.1538) (-55.8117, 9.0134) (-55.8092, 8.8718) (-55.8215, 8.7306) (-55.8493, 8.5918) (-55.8859, 8.4551) (-55.935, 8.3224) (-55.9905, 8.1923) (-56.0768, 8.0245) (-56.152, 7.9047) (-56.2022, 7.8249) knots 0 0 0 0 0.062498 0.093754 0.125008 0.156267 0.187517 0.21877 0.250029 0.281282 0.312529 0.343776 0.37503 0.406277 0.437515 0.468744 0.5 0.531256 0.562485 0.593723 0.62497 0.656224 0.687471 0.718718 0.749971 0.78123 0.812483 0.843733 0.874992 0.906246 0.937502 1 1 1 1 construction
  spline S102 degree 3 poles (-56.2022, 7.8249) (-56.2307, 7.7646) (-56.2877, 7.644) (-56.35, 7.4537) (-56.4034, 7.261) (-56.4612, 7.0007) (-56.5134, 6.6712) (-56.5488, 6.2727) (-56.5607, 5.8728) (-56.551, 5.4729) (-56.5232, 5.0737) (-56.4894, 4.8092) (-56.4724, 4.677) knots 0 0 0 0 0.062465 0.124964 0.187468 0.249973 0.374966 0.499967 0.624972 0.749981 0.874991 1 1 1 1 construction
  arc A32 (-56.4724, 4.677) -> (-55.2721, 4.146) centre (-49, 19.9467) ccw construction
  spline S103 degree 3 poles (-55.2721, 4.146) (-55.1629, 4.2225) (-54.9444, 4.3753) (-54.6304, 4.6233) (-54.3279, 4.8851) (-54.04, 5.1629) (-53.769, 5.4572) (-53.5603, 5.7174) (-53.4066, 5.9353) (-53.2999, 6.1044) (-53.2009, 6.2785) (-53.1501, 6.4018) (-53.1247, 6.4635) knots 0 0 0 0 0.125009 0.250019 0.375028 0.500033 0.625034 0.750027 0.812532 0.875036 0.937535 1 1 1 1 construction
  spline S104 degree 3 poles (-53.1247, 6.4635) (-53.0993, 6.5543) (-53.0613, 6.6905) (-52.9952, 6.8672) (-52.9363, 6.9959) (-52.8711, 7.1215) (-52.7945, 7.2405) (-52.7105, 7.3544) (-52.6144, 7.4585) (-52.5079, 7.5519) (-52.3907, 7.6317) (-52.2639, 7.6952) (-52.1293, 7.7402) (-51.9895, 7.7643) (-51.8475, 7.767) (-51.7075, 7.7447) (-51.5699, 7.7127) (-51.431, 7.6866) (-51.2939, 7.6506) (-51.1649, 7.5911) (-51.0466, 7.5128) (-50.9416, 7.4174) (-50.8511, 7.3082) (-50.7759, 7.1881) (-50.716, 7.0597) (-50.6698, 6.9257) (-50.6387, 6.7876) (-50.6165, 6.6479) (-50.6074, 6.5066) (-50.6052, 6.3652) (-50.6158, 6.1768) (-50.6358, 6.0368) (-50.6492, 5.9434) knots 0 0 0 0 0.062498 0.093754 0.125008 0.156267 0.187517 0.21877 0.250029 0.281282 0.312529 0.343776 0.37503 0.406277 0.437515 0.468744 0.5 0.531256 0.562485 0.593723 0.62497 0.656224 0.687471 0.718718 0.749971 0.78123 0.812483 0.843733 0.874992 0.906246 0.937502 1 1 1 1 construction
  spline S105 degree 3 poles (-50.6492, 5.9434) (-50.6507, 5.8768) (-50.6537, 5.7435) (-50.6332, 5.5442) (-50.6036, 5.3465) (-50.5505, 5.0851) (-50.4642, 4.763) (-50.3345, 4.3845) (-50.1827, 4.0143) (-50.0111, 3.6529) (-49.8234, 3.2996) (-49.6849, 3.0717) (-49.6157, 2.9578) knots 0 0 0 0 0.062465 0.124964 0.187468 0.249973 0.374966 0.499967 0.624972 0.749981 0.874991 1 1 1 1 construction
  arc A33 (-49.6157, 2.9578) -> (-48.3032, 2.961) centre (-49, 19.9467) ccw construction
  spline S106 degree 3 poles (-48.3032, 2.961) (-48.2345, 3.0752) (-48.097, 3.3037) (-47.911, 3.6579) (-47.7412, 4.0201) (-47.5912, 4.391) (-47.4632, 4.7701) (-47.3785, 5.0927) (-47.3267, 5.3543) (-47.298, 5.5522) (-47.2784, 5.7515) (-47.2821, 5.8848) (-47.2839, 5.9515) knots 0 0 0 0 0.125009 0.250019 0.375028 0.500033 0.625034 0.750027 0.812532 0.875036 0.937535 1 1 1 1 construction
  spline S107 degree 3 poles (-47.2839, 5.9515) (-47.2978, 6.0448) (-47.3185, 6.1847) (-47.3299, 6.373) (-47.3284, 6.5145) (-47.32, 6.6557) (-47.2984, 6.7956) (-47.268, 6.9339) (-47.2225, 7.068) (-47.1632, 7.1967) (-47.0886, 7.3172) (-46.9986, 7.4268) (-46.894, 7.5227) (-46.7761, 7.6016) (-46.6474, 7.6617) (-46.5105, 7.6983) (-46.3717, 7.7251) (-46.2342, 7.7578) (-46.0943, 7.7807) (-45.9523, 7.7788) (-45.8124, 7.7553) (-45.6776, 7.7109) (-45.5505, 7.648) (-45.4329, 7.5688) (-45.326, 7.4759) (-45.2293, 7.3723) (-45.1448, 7.2588) (-45.0677, 7.1401) (-45.0018, 7.0148) (-44.9424, 6.8865) (-44.8754, 6.7101) (-44.8367, 6.574) (-44.811, 6.4833) knots 0 0 0 0 0.062498 0.093754 0.125008 0.156267 0.187517 0.21877 0.250029 0.281282 0.312529 0.343776 0.37503 0.406277 0.437515 0.468744 0.5 0.531256 0.562485 0.593723 0.62497 0.656224 0.687471 0.718718 0.749971 0.78123 0.812483 0.843733 0.874992 0.906246 0.937502 1 1 1 1 construction
  spline S108 degree 3 poles (-44.811, 6.4833) (-44.7852, 6.4218) (-44.7338, 6.2988) (-44.634, 6.1251) (-44.5265, 5.9565) (-44.3718, 5.7393) (-44.1619, 5.4801) (-43.8894, 5.1871) (-43.6001, 4.9107) (-43.2965, 4.6503) (-42.9813, 4.4039) (-42.7621, 4.2521) (-42.6524, 4.1762) knots 0 0 0 0 0.062465 0.124964 0.187468 0.249973 0.374966 0.499967 0.624972 0.749981 0.874991 1 1 1 1 construction
  arc A34 (-42.6524, 4.1762) -> (-41.4547, 4.7129) centre (-49, 19.9467) ccw construction
  circle A35 centre (-49, 19.9467) radius 1.1 construction
  line L25 (-111, -304.8) -> (-111, 304.8) construction
  line L26 (64.1879, 304.8) -> (-111, 304.8) construction
  line L27 (64.1879, -304.8) -> (64.1879, 304.8) construction
  line L28 (-111, -304.8) -> (64.1879, -304.8) construction
  line L29 (-63, 33.9467) -> (57.1879, 33.9467)
  line L30 (57.1879, 33.9467) -> (57.1879, -21.0467)
  line L31 (57.1879, -21.0467) -> (-63, -21.0467)
  line L32 (-63, -21.0467) -> (-63, 33.9467)
  line L33 (64.1879, -304.8) -> (64.1879, 304.8) construction
  line L34 (57.1879, 304.8) -> (64.1879, 304.8) construction
  line L35 (57.1879, -304.8) -> (57.1879, 304.8) construction
  line L36 (64.1879, -304.8) -> (57.1879, -304.8) construction
  arc A36 (-41.35, 26.5031) -> (-56.65, 26.5031) centre (-49, 19.8323) ccw
  line L37 (-56.65, 26.5031) -> (-56.65, 13.3902)
  arc A37 (-56.65, 13.3902) -> (-41.35, 13.3902) centre (-49, 20.0611) ccw
  line L38 (-41.35, 13.3902) -> (-41.35, 26.5031)
  arc A38 (-6.4, 26.4844) -> (-21.6, 26.4844) centre (-14, 19.8323) ccw
  line L39 (-21.6, 26.4844) -> (-21.6, 13.409)
  arc A39 (-21.6, 13.409) -> (-6.4, 13.409) centre (-14, 20.0611) ccw
  line L40 (-6.4, 13.409) -> (-6.4, 26.4844)
  line L41 (-63, -6.0467) -> (57.1879, -6.0467)
  circle A40 centre (-14, 19.9467) radius 17 construction
  line L42 (57.1879, 6.9467) -> (-63, 6.9467)
  circle A41 centre (-49, 19.9467) radius 17 construction
  circle A42 centre (-14, 19.9467) radius 19
  circle A43 centre (-49, 19.9467) radius 19
  line L43 (-57.7, 17.9164) -> (-57.7, 21.977) construction
  arc A44 (-57.7, 17.9164) -> (-56.5, 16.4467) centre (-56.2, 17.9164) ccw construction
  line L44 (-56.5, 23.4467) -> (-56.5, 16.4467) construction
  arc A45 (-56.5, 23.4467) -> (-57.7, 21.977) centre (-56.2, 21.977) ccw construction
  line L45 (-56.8008, 23.3514) -> (-56.8008, 26.9467) construction
  line L46 (-56.8008, 26.9467) -> (-57, 26.9467) construction
  line L47 (-57, 23.2458) -> (-57, 26.9467) construction
  arc A46 (-56.8008, 23.3514) -> (-57, 23.2458) centre (-56.2, 21.977) ccw
  line L48 (-57, 27.9467) -> (-57, 26.9467) construction
  line L49 (-56.8008, 26.9467) -> (-56.8008, 27.9467) construction
  line L50 (-56.8008, 11.9467) -> (-56.8008, 12.9467) construction
  line L51 (-57, 12.9467) -> (-57, 11.9467) construction
  line L52 (-57, 12.9467) -> (-57, 16.6475) construction
  line L53 (-56.8008, 12.9467) -> (-56.8008, 16.5419) construction
  line L54 (-5.3, 21.977) -> (-5.3, 17.9164) construction
  arc A47 (-5.3, 21.977) -> (-6.5, 23.4467) centre (-6.8, 21.977) ccw construction
  line L55 (-6.5, 16.4467) -> (-6.5, 23.4467) construction
  arc A48 (-6.5, 16.4467) -> (-5.3, 17.9164) centre (-6.8, 17.9164) ccw construction
  line L56 (-6, 26.9467) -> (-6, 23.2458) construction
  line L57 (-6, 26.9467) -> (-6.1992, 26.9467) construction
  line L58 (-6.1992, 26.9467) -> (-6.1992, 23.3514) construction
  arc A49 (-6, 23.2458) -> (-6.1992, 23.3514) centre (-6.8, 21.977) ccw
  arc A50 (-12.4, 10.1899) -> (-6.5, 13.4467) centre (-14, 20.0611) ccw construction
  arc A51 (-12.4, 10.1899) -> (-15.6, 10.1899) centre (-14, 10.193) ccw construction
  arc A52 (-21.5, 13.4467) -> (-15.6, 10.1899) centre (-14, 20.0611) ccw construction
  line L59 (-21.5, 13.4467) -> (-21.5, 26.4467) construction
  arc A53 (-15.5844, 29.706) -> (-21.5, 26.4467) centre (-14, 19.8323) ccw construction
  arc A54 (-15.5844, 29.706) -> (-12.4156, 29.706) centre (-14, 29.9292) ccw construction
  arc A55 (-6.5, 26.4467) -> (-12.4156, 29.706) centre (-14, 19.8323) ccw construction
  line L60 (-6.5, 26.4467) -> (-6.5, 13.4467) construction
  arc A56 (-10.5, 23.5174) -> (-10.5, 16.376) centre (-14, 19.9467) ccw construction
  line L61 (-10.5, 16.376) -> (-10.5, 23.5174) construction
  line L62 (-6, 26.9467) -> (-6, 27.9467) construction
  line L63 (-6.1992, 27.9467) -> (-6.1992, 26.9467) construction
  line L64 (-6.1992, 12.9467) -> (-6.1992, 11.9467) construction
  line L65 (-6, 11.9467) -> (-6, 12.9467) construction
  line L66 (-57.85, 21.977) -> (-57.85, 17.9164) construction
  arc A57 (-57.85, 17.9164) -> (-56.35, 16.2732) centre (-56.2, 17.9164) ccw construction
  line L67 (-56.35, 16.2732) -> (-56.35, 23.6202) construction
  arc A58 (-56.35, 23.6202) -> (-57.85, 21.977) centre (-56.2, 21.977) ccw construction
  line L68 (-49, 19.9467) -> (-14, 19.9467) construction
  line L69 (-31.5, 19.9467) -> (-31.5, 26.6799) construction
  line L70 (-49.025, 23.3133) -> (-49.025, 13.9899) construction
  line L71 (0, 304.8) -> (0, -304.8)
  line L72 (-62.3, -13.4767) -> (-62.3, -10.4767) construction
  line L73 (-62.3, -13.4767) -> (-56.8, -13.4767) construction
  line L74 (-56.8, -10.4767) -> (-56.8, -13.4767) construction
  line L75 (-61.4, -10.4767) -> (-56.8, -10.4767) construction
  line L76 (-62.3, -10.4767) -> (-61.4, -10.4767) construction
  line L77 (-62.3, -16.4767) -> (-62.3, -13.4767) construction
  line L78 (-62.3, -16.4767) -> (-56.8, -16.4767) construction
  line L79 (-56.8, -13.4767) -> (-56.8, -16.4767) construction
  line L80 (-61.4, -13.4767) -> (-56.8, -13.4767) construction
  line L81 (-62.3, -13.4767) -> (-61.4, -13.4767) construction
  arc A59 (-5.15, 21.977) -> (-6.65, 23.6202) centre (-6.8, 21.977) ccw construction
  line L82 (-5.15, 21.977) -> (-5.15, 17.9164) construction
  arc A60 (-6.65, 16.2732) -> (-5.15, 17.9164) centre (-6.8, 17.9164) ccw construction
  line L83 (-6.65, 16.2732) -> (-6.65, 23.6202) construction
  line L84 (-6, 27.9467) -> (-6.1992, 27.9467) construction
  line L85 (-6.1992, 11.9467) -> (-6, 11.9467) construction
  line L86 (-6, 16.6475) -> (-6, 12.9467) construction
  line L87 (-6.1992, 16.5419) -> (-6.1992, 12.9467) construction
  line L88 (-57, 11.9467) -> (-56.8008, 11.9467) construction
  line L89 (-56.8008, 27.9467) -> (-57, 27.9467) construction
  line L90 (-14, 19.9467) -> (-14, 23.6202) construction
  line L91 (-22, 26.9467) -> (-22, 23.2458) construction
  line L92 (-21.8008, 26.9467) -> (-21.8008, 23.3514) construction
  line L93 (-22, 26.9467) -> (-22, 27.9467) construction
  line L94 (-21.8008, 27.9467) -> (-21.8008, 26.9467) construction
  line L95 (-21.8008, 12.9467) -> (-21.8008, 11.9467) construction
  line L96 (-22, 11.9467) -> (-22, 12.9467) construction
  arc A61 (-21.35, 23.6202) -> (-22.85, 21.977) centre (-21.2, 21.977) ccw construction
  line L97 (-22.85, 21.977) -> (-22.85, 17.9164) construction
  arc A62 (-22.85, 17.9164) -> (-21.35, 16.2732) centre (-21.2, 17.9164) ccw construction
  line L98 (-22, 27.9467) -> (-21.8008, 27.9467) construction
  line L99 (-21.8008, 11.9467) -> (-22, 11.9467) construction
  line L100 (-22, 16.6475) -> (-22, 12.9467) construction
  line L101 (-21.8008, 16.5419) -> (-21.8008, 12.9467) construction
  line L102 (-19.806, 28.0967) -> (-24.85, 28.0967)
  line L103 (-24.85, 28.0967) -> (-24.85, 11.7967)
  line L104 (-24.85, 11.7967) -> (-19.806, 11.7967)
  line L105 (-19.806, 11.7967) -> (-19.806, 28.0967) construction
  spline S109 degree 4 poles (-36.035, 25.4891) (-36.2337, 25.4145) (-36.4654, 25.3084) (-36.7493, 25.1259) (-37.0078, 24.8408) (-37.143, 24.6066) (-37.2101, 24.3458) (-37.2134, 24.086) (-37.1054, 23.8115) (-37.0314, 23.5259) (-36.8761, 23.3177) (-36.6685, 23.1461) (-36.4214, 23.0361) (-36.0447, 22.9573) (-35.7078, 22.9766) (-35.4579, 23.027) (-35.2533, 23.0834) knots 0 0 0 0 0 0.162655 0.224844 0.286017 0.346335 0.407305 0.469139 0.53086 0.592695 0.653664 0.713983 0.775156 0.837344 1 1 1 1 1 construction
  line L106 (-43.194, 28.0967) -> (-38.15, 28.0967)
  line L107 (-38.15, 28.0967) -> (-38.15, 11.7967)
  line L108 (-38.15, 11.7967) -> (-43.194, 11.7967)
  point P0 (0, 0)
  point P1 (-55.0975, 27.9467)
  point P2 (-31.5, 12.5474)
  point P3 (-35.1436, 6.9467)
  point P4 (-27.8564, 6.9467)
  point P5 (-62.8564, 6.9467)
  point P6 (-31.5, 27.346)
  point P7 (-0.1436, 6.9467)
  point P8 (0, 7.1014)
  point P9 (0, 32.7919)
  point P10 (0, 33.9467)
  point P11 (0, -21.0467)
  point P12 (0, -6.0467)
  point P13 (-36.3409, 25.3578)
  point P14 (-36.5963, 25.2099)
  point P15 (-36.8201, 25.0333)
  point P16 (-37.0009, 24.8299)
  point P17 (-37.1299, 24.5989)
  point P18 (-37.1963, 24.3487)
  point P19 (-37.1926, 24.0938)
  point P20 (-37.1118, 23.8094)
  point P21 (-37.01, 23.5318)
  point P22 (-36.8632, 23.3234)
  point P23 (-36.6624, 23.16)
  point P24 (-36.4222, 23.049)
  point P25 (-36.1564, 22.9907)
  point P26 (-35.8716, 22.9794)
  point P27 (-35.578, 23.0098)
  point P28 (-43.1074, 28.0967)
  point P29 (-43.1074, 11.7967)
  dimension "d88" = 1
  dimension "d90" = 1
  dimension "d91" = 0.75
  dimension "d92" = 1
  dimension "d14" = 14
  dimension "d15" = 14
  dimension "d16" = 0.15
  dimension "d17" = 0.1
  dimension "d18" = 0.1
  dimension "d19" = 1
  dimension "d20" = 2
  dimension "d21" = 2
  dimension "d22" = 0.15
  dimension "d65" = 0.15
  dimension "d66" = 0.15
  dimension "d67" = 2
  dimension "d68" = 15
  constraints: 86 end point, 24 symmetric about line, 23 point on circle, 12 centre point, 7 horizontal, 5 perpendicular, 5 vertical, 4 point on line, 3 parallel, 2 coincident, 1 collinear, 1 midpoint, 51 other
  measures "d14" distance from line of A4.centre L29
  measures "d15" distance from line of A24.centre L32
  measures "d16" distance between parallel lines of L24 L38
  measures "d17" distance between parallel lines of L21 L40
  measures "d18" distance between parallel lines of L19 L41
  measures "d19" distance from line of L7.start L42
  measures "d22" radial gap between concentric circles of A45 A58
  measures "d65" radial gap between concentric circles of A47 A59
  measures "d66" distance between parallel lines of L99 L104
  measures "d67" distance between parallel lines of L97 L103
  measures "d68" distance between parallel lines of L41 L31
extrude "Extrusion3" add sketch "Sketch2" against normal blind 28.25 contours L29 A43 L32 | L29 A43 A42 L42 L32 | L29 A42 A43 | A43 L42 L32 | L29 A42 L71 L42 A43 | A43 A42 | L42 A43 A42 L71 L41 L32 | L42 A43 | L29 L71 A42 | A42 L42 A43 | L41 L71 L31 L32 | L42 A42 | L71 L42 A42
extrude "Extrusion4" add sketch "Sketch2" along normal blind 11 contours L41 L71 L31 L32
sketch "Sketch6" plane through (0, -33.9467, 0) normal (0, -1, 0) x (1, 0, 0)
  line L0 (0, 0) -> (-9.9035, 0) projected
  line L1 (-9.9035, 0) -> (-9.9035, -0.8852) projected
  spline S0 degree 4 poles (-9.9035, -0.8852) (-13.0419, -1.1842) (-21.2538, 1.0327) (-27.8606, -5.346) (-33.2586, -4.0317) (-34.8616, -3.7545) knots 0 0 0 0 0 0.558486 0.866888 0.866888 0.866888 0.866888 0.866888 projected
  line L2 (-34.8616, -3.7545) -> (-37.2153, -3.929) projected
  line L3 (-37.2153, -3.929) -> (-37.2153, -4.9671) projected
  line L4 (-37.2153, -4.9671) -> (-41.1207, -5.3635) projected
  spline S1 degree 2 poles (-41.1207, -5.3635) (-45.6353, -4.1273) (-50.1475, -5.6677) knots 0 0 0 1 1 1 projected
  spline S2 degree 2 poles (-50.1475, -5.6677) (-53.2023, -5.0279) (-57.1879, -6.1401) knots 0 0 0 1 1 1 projected
  line L5 (-57.1879, -6.1401) -> (-57.1879, -13.1401) projected
  line L6 (-57.1879, -13.1401) -> (-64.1879, -13.1401) projected
  line L7 (-64.1879, -13.1401) -> (-64.1879, -28.5) projected
  line L8 (-64.1879, -28.5) -> (111, -28.5) projected
  line L9 (111, -28.5) -> (111, -18.5) projected
  line L10 (111, -18.5) -> (0, -18.5) projected
  line L11 (0, -18.5) -> (0, 0) projected
extrude "Extrusion7" cut sketch "Sketch6" against normal through all
ref_plane "Work Plane2" through (42.85, 5.9467, -5) normal (0, 0, 1) x (0, -1, 0)